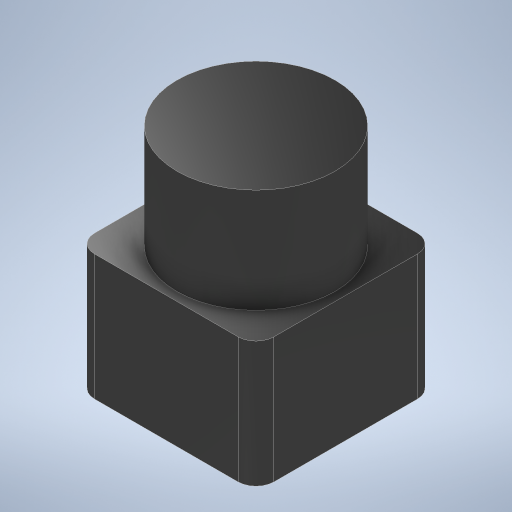
# Autodesk Inventor part: LiDAR_un
Saved by Autodesk Inventor 2023 (Build 270158000, 158)
## iProperties
Created: 2023-03-18
Part Number: LiDAR_un
Material: ABS プラスチック
Document SubType Name: Modeling
Designer: mkhr7
Density: 1.06 g/cm^3
Appearance: 光沢 - 黒
Author: mkhr7
Autodesk Inventor part; units mm, degrees
ref_plane "YZ Plane" through (0, 0, 0) normal (1, 0, 0) x (0, 1, 0)
ref_plane "XZ Plane" through (0, 0, 0) normal (0, 1, 0) x (-1, 0, 0)
ref_plane "XY Plane" through (0, 0, 0) normal (0, 0, 1) x (1, 0, 0)
sketch "スケッチ1" plane through (0, 0, 0) normal (0, 1, 0) x (-1, 0, 0)
  line L0 (0, 0) -> (50, 0)
  line L1 (50, 0) -> (50, -50)
  line L2 (50, -50) -> (0, -50)
  line L3 (0, -50) -> (0, 0)
  dimension "d0" = 50
  dimension "d1" = 50
  constraints: 8 end point, 2 parallel, 1 horizontal, 1 perpendicular
  measures "d0" distance of L1.end L2.end
  measures "d1" distance of L0.end L1.end
extrude "押し出し1" add sketch "スケッチ1" along normal blind 35
sketch "スケッチ2" plane through (0, 35, 0) normal (0, 1, 0) x (1, 0, 0)
  circle A0 centre (-24.4444, 24.4444) radius 22
  point P0 (0, 0)
  dimension "d4" = 44
  constraints: 1 centre point
  measures "d4" diameter of A0
extrude "押し出し2" add sketch "スケッチ2" along normal blind 29
fillet "フィレット1" radius 5 4 edges at (-50, 17.5, 0) (0, 17.5, 0) (0, 17.5, -50) (-50, 17.5, -50)
sketch "スケッチ3" plane through (0, 0, 0) normal (0, -1, 0) x (1, 0, 0)
  arc A0 (-50, -45) -> (-45, -50) centre (-45, -45) ccw projected
  line L0 (-5, -50) -> (-45, -50) projected
  arc A1 (-5, -50) -> (0, -45) centre (-5, -45) ccw projected
  line L1 (0, -5) -> (0, -45) projected
  arc A2 (0, -5) -> (-5, 0) centre (-5, -5) ccw projected
  line L2 (-45, 0) -> (-5, 0) projected
  arc A3 (-45, 0) -> (-50, -5) centre (-45, -5) ccw projected
  line L3 (-50, -45) -> (-50, -5) projected
  point P0 (0, 0)
  constraints: 4 coincident
hole "穴1" at (-5, 0, -5) at (-5, 0, -45) at (-45, 0, -45) at (-45, 0, -5) direction (0, 1, 0) diameter 3.1 depth 8 tip angle 118
